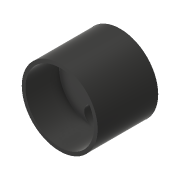
# Autodesk Inventor part: Cap Cap no LED
Saved by Autodesk Inventor 2017 (Build 210142000, 142)
## iProperties
Created: 2016-08-05
Part Number: Cap Cap no LED
Material: Generic
Document SubType Name: Modeling
Designer: ge937963
Density: 1 g/cm^3
Appearance: Smooth - Black
Mass: 3.1063 g
Surface Area: 31.3911 cm^2
Volume: 3.1063 cm^3
Author: ge937963
Autodesk Inventor part; units mm, degrees
ref_plane "YZ Plane" through (0, 0, 0) normal (1, 0, 0) x (0, 1, 0)
ref_plane "XZ Plane" through (0, 0, 0) normal (0, 1, 0) x (-1, 0, 0)
sketch "Sketch1" plane through (0, 0, 0) normal (0, 0, 1) x (1, 0, 0)
  circle A0 centre (0, 0) radius 9.025
  dimension "d0" = 18.05
  constraints: 1 centre point, 1 coincident
  measures "d0" diameter of A0
extrude "Extrusion1" add sketch "Sketch1" along normal blind 6.35
sketch "Sketch4" plane through (0, 0, 6.35) normal (0, 0, 1) x (1, 0, 0)
  circle A0 centre (0, 0) radius 3.175
  dimension "d6" = 6.35
  constraints: 1 centre point, 1 coincident
  measures "d6" diameter of A0
sketch "Sketch6" plane through (0, 0, 6.35) normal (0, 0, 1) x (1, 0, 0)
  circle A0 centre (0, 0) radius 9.025
  circle A1 centre (0, 0) radius 8.2312
  circle A2 centre (0, 0) radius 9.025 projected
  dimension "d11" = 0.7937
  constraints: 2 centre point, 2 coincident, 1 concentric
  measures "d11" radial gap between concentric circles of A0 A1
ref_plane "Work Plane1" through (-9.0805, -9.0805, 27.1559) normal (0, 0, -1) x (0.0062, 1, 0)
extrude "Extrusion3" add sketch "Sketch6" along normal up to surface (20.8059 mm away)
sketch "Sketch7" plane through (0, 0, 6.35) normal (0, 0, 1) x (1, 0, 0)
  circle A0 centre (0, 5.9436) radius 1.397
  circle A1 centre (0, -5.9436) radius 1.397
  circle A2 centre (0, 0) radius 8.2312 projected
  dimension "d20" = 2.794
  dimension "d21" = 2.794
  dimension "d22" = 5.9436
  dimension "d23" = 5.9436
  constraints: 2 centre point
  measures "d20" diameter of A0
  measures "d21" diameter of A1
  measures "d22" distance of A2.centre A1.centre
  measures "d23" distance of point (0, 0) A0.centre
extrude "Extrusion4" cut sketch "Sketch7" against normal blind 25.4 contours A0 | A1
sketch "Sketch8" plane through (0, 0, 6.35) normal (0, 0, 1) x (1, 0, 0)
  circle A0 centre (0, 5.9436) radius 2.286
  circle A1 centre (0, -5.9436) radius 2.286
  circle A2 centre (0, 5.9436) radius 1.397 projected
  circle A3 centre (0, -5.9436) radius 1.397 projected
  point P0 (0, 0)
  dimension "d16" = 4.572
  dimension "d17" = 4.572
  constraints: 2 centre point, 2 concentric, 2 vertical alignment
  measures "d16" diameter of A0
  measures "d17" diameter of A1
extrude "Extrusion5" cut sketch "Sketch8" against normal blind 4.7625 contours A0 | A1 | A2 | A3
extrude "Extrusion6" cut sketch "Sketch4" against normal blind 25.4
sketch "Sketch9" plane through (0, 0, 27.1559) normal (0, 0, 1) x (1, 0, 0)
  circle A0 centre (27.8867, -20.1987) radius 65.8542
  point P0 (0, 0)
  constraints: 1 centre point
extrude "Extrusion7" cut sketch "Sketch9" against normal blind 12.7
body "Solid1"
